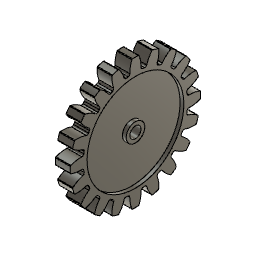
spur gear v1 (Autodesk Fusion 360 design; units mm, degrees)
Autodesk Fusion 360 part; units mm, degrees
sketch "Sketch1" plane through (0, 0, 0) normal (1, 0, 0) x (0, 1, 0)
  line L0 (0, 0) -> (0, 17.1609) construction
  line L1 (0, 0) -> (16.4802, 0) construction
  line L2 (0, 0) -> (1.095, 6.9138)
  arc A0 (0.7464, 7.1896) -> (0.4825, 8.6787) centre (-2.8935, 7.3125) ccw
  arc A1 (0.3944, 8.7411) -> (-0.3944, 8.7411) centre (0, 0) ccw
  arc A2 (0.6886, 7.9703) -> (8, 0) centre (0, 0) ccw
  arc A3 (1.095, 6.9138) -> (0.9619, 6.9336) centre (0, 0) ccw
  arc A4 (0.7464, 7.1896) -> (0.9619, 6.9336) centre (0.9963, 7.1812) ccw
  arc A5 (0.4825, 8.6787) -> (0.3944, 8.7411) centre (0.3898, 8.6412) ccw
  arc A6 (-0.3944, 8.7411) -> (-0.4825, 8.6787) centre (-0.3898, 8.6412) ccw
  arc A7 (-0.4825, 8.6787) -> (-0.7464, 7.1896) centre (2.8935, 7.3125) ccw
  arc A8 (-0.9619, 6.9336) -> (-0.7464, 7.1896) centre (-0.9963, 7.1812) ccw
  line L3 (0, 0) -> (-1.095, 6.9138)
  arc A9 (-0.9619, 6.9336) -> (-1.095, 6.9138) centre (0, 0) ccw
  dimension "d1" = 14
  dimension "d2" = 16
  dimension "d3" = 17.5
  dimension "d6" = 9
  dimension "d7" = 0.25
  dimension "d8" = 0.1
  constraint coincident L0.start L1.start
  constraint concentric A1 A3
  constraint vertical L0
  constraint perpendicular L0 L1
  constraint coincident L1 A2.end
  constraint coincident A0 A2.start
  constraint tangent A0 A4
  constraint tangent A3 A4
  constraint tangent A1 A5
  constraint tangent A0 A5
  constraint symmetric L0 L1.start L2.start
  constraint symmetric L0 A0 A7
  constraint symmetric L0 L2.end L3.end
  constraint symmetric L0 A3 A9
  constraint symmetric L0 A0.start A7.end
  constraint symmetric L0 A3.end A8.start
  constraint symmetric L0 A4 A8
  constraint symmetric L0 A1.start A1.end
  constraint symmetric L0 A0.end A6.end
  constraint symmetric L0 A5 A6
  measures "d1" diameter of A3
  measures "d2" diameter of A2
  measures "d3" diameter of A1
  measures "d6" angle of L0 L2
  measures "d7" radius of A4
  measures "d8" radius of A5
extrude "Extrude1" add sketch "Sketch1" along normal blind 2 makes body 1
pattern_circular "C-Pattern1" count 20 over 360 about axis through (1.75, 0, 0) along (1, 0, 0) of bodies 1 makes body 2 at (0.6667, -0.365, 2.3046) makes body 3 at (0, -2.72, 3.7437) makes body 4 at (0, -3.7437, 2.72) makes body 5 at (0, -4.401, 1.43) makes body 6 at (0, -4.6275, 0) makes body 7 at (0, -4.401, -1.43) makes body 8 at (0, -3.7437, -2.72) makes body 9 at (0, -2.72, -3.7437) makes body 10 at (0, -1.43, -4.401) makes body 11 at (0, 0, -4.6275) makes body 12 at (0, 1.43, -4.401) makes body 13 at (0, 2.72, -3.7437) makes body 14 at (0, 3.7437, -2.72) makes body 15 at (0, 4.401, -1.43) makes body 16 at (0, 4.6275, 0) makes body 17 at (0, 4.401, 1.43) makes body 18 at (0, 3.7437, 2.72) makes body 19 at (0, 2.72, 3.7437) makes body 20 at (0.6667, 0.365, 2.3046)
combine "Combine1" operation add target body 19 tool bodies 18 17 16 14 15 13 12 11 10 9 8 7 6 5 4 3 2 1 20
sketch "Sketch2" plane through (2, 0, 0) normal (1, 0, 0) x (0, 1, 0)
  arc A0 (5.3778, -4.8299) -> (6.7376, -5.4916) centre (7.6167, -1.9573) ccw
  arc A1 (6.7376, -5.4916) -> (6.8399, -5.4569) centre (6.7617, -5.3946) ccw
  arc A2 (6.8399, -5.4569) -> (7.3035, -4.8189) centre (0, 0) ccw
  arc A3 (7.3035, -4.8189) -> (7.3049, -4.7108) centre (7.22, -4.7638) ccw
  arc A4 (7.3049, -4.7108) -> (6.2553, -3.6221) centre (4.2152, -6.6391) ccw
  arc A5 (6.1748, -3.2972) -> (6.2553, -3.6221) centre (6.3953, -3.415) ccw
  arc A6 (6.1748, -3.2972) -> (6.297, -3.0575) centre (0, 0) ccw
  arc A7 (6.6071, -2.9316) -> (6.297, -3.0575) centre (6.5219, -3.1667) ccw
  arc A8 (6.6071, -2.9316) -> (8.1048, -3.1408) centre (7.8487, 0.4922) ccw
  arc A9 (8.1048, -3.1408) -> (8.1914, -3.0762) centre (8.0978, -3.041) ccw
  arc A10 (8.1914, -3.0762) -> (8.4351, -2.3261) centre (0, 0) ccw
  arc A11 (8.4351, -2.3261) -> (8.4031, -2.2229) centre (8.3387, -2.2995) ccw
  arc A12 (8.4031, -2.2229) -> (7.0684, -1.5118) centre (6.0604, -5.0116) ccw
  arc A13 (6.8915, -1.2277) -> (7.0684, -1.5118) centre (7.1376, -1.2716) ccw
  arc A14 (6.8915, -1.2277) -> (6.9336, -0.9619) centre (0, 0) ccw
  arc A15 (7.1896, -0.7464) -> (6.9336, -0.9619) centre (7.1812, -0.9963) ccw
  arc A16 (7.1896, -0.7464) -> (8.6787, -0.4825) centre (7.3125, 2.8935) ccw
  arc A17 (8.6787, -0.4825) -> (8.7411, -0.3944) centre (8.6412, -0.3898) ccw
  arc A18 (8.7411, -0.3944) -> (8.7411, 0.3944) centre (0, 0) ccw
  arc A19 (8.7411, 0.3944) -> (8.6787, 0.4825) centre (8.6412, 0.3898) ccw
  arc A20 (8.6787, 0.4825) -> (7.1896, 0.7464) centre (7.3125, -2.8935) ccw
  arc A21 (6.9336, 0.9619) -> (7.1896, 0.7464) centre (7.1812, 0.9963) ccw
  arc A22 (6.9336, 0.9619) -> (6.8915, 1.2277) centre (0, 0) ccw
  arc A23 (7.0684, 1.5118) -> (6.8915, 1.2277) centre (7.1376, 1.2716) ccw
  arc A24 (7.0684, 1.5118) -> (8.4031, 2.2229) centre (6.0604, 5.0116) ccw
  arc A25 (8.4031, 2.2229) -> (8.4351, 2.3261) centre (8.3387, 2.2995) ccw
  arc A26 (8.4351, 2.3261) -> (8.1914, 3.0762) centre (0, 0) ccw
  arc A27 (8.1914, 3.0762) -> (8.1048, 3.1408) centre (8.0978, 3.041) ccw
  arc A28 (8.1048, 3.1408) -> (6.6071, 2.9316) centre (7.8487, -0.4922) ccw
  arc A29 (6.297, 3.0575) -> (6.6071, 2.9316) centre (6.5219, 3.1667) ccw
  arc A30 (6.297, 3.0575) -> (6.1748, 3.2972) centre (0, 0) ccw
  arc A31 (6.2553, 3.6221) -> (6.1748, 3.2972) centre (6.3953, 3.415) ccw
  arc A32 (6.2553, 3.6221) -> (7.3049, 4.7108) centre (4.2152, 6.6391) ccw
  arc A33 (7.3049, 4.7108) -> (7.3035, 4.8189) centre (7.22, 4.7638) ccw
  arc A34 (7.3035, 4.8189) -> (6.8399, 5.4569) centre (0, 0) ccw
  arc A35 (6.8399, 5.4569) -> (6.7376, 5.4916) centre (6.7617, 5.3946) ccw
  arc A36 (6.7376, 5.4916) -> (5.3778, 4.8299) centre (7.6167, 1.9573) ccw
  arc A37 (5.044, 4.8537) -> (5.3778, 4.8299) centre (5.2241, 5.027) ccw
  arc A38 (5.044, 4.8537) -> (4.8537, 5.044) centre (0, 0) ccw
  arc A39 (4.8299, 5.3778) -> (4.8537, 5.044) centre (5.027, 5.2241) ccw
  arc A40 (4.8299, 5.3778) -> (5.4916, 6.7376) centre (1.9573, 7.6167) ccw
  arc A41 (5.4916, 6.7376) -> (5.4569, 6.8399) centre (5.3946, 6.7617) ccw
  arc A42 (5.4569, 6.8399) -> (4.8189, 7.3035) centre (0, 0) ccw
  arc A43 (4.8189, 7.3035) -> (4.7108, 7.3049) centre (4.7638, 7.22) ccw
  arc A44 (4.7108, 7.3049) -> (3.6221, 6.2553) centre (6.6391, 4.2152) ccw
  arc A45 (3.2972, 6.1748) -> (3.6221, 6.2553) centre (3.415, 6.3953) ccw
  arc A46 (3.2972, 6.1748) -> (3.0575, 6.297) centre (0, 0) ccw
  arc A47 (2.9316, 6.6071) -> (3.0575, 6.297) centre (3.1667, 6.5219) ccw
  arc A48 (2.9316, 6.6071) -> (3.1408, 8.1048) centre (-0.4922, 7.8487) ccw
  arc A49 (3.1408, 8.1048) -> (3.0762, 8.1914) centre (3.041, 8.0978) ccw
  arc A50 (3.0762, 8.1914) -> (2.3261, 8.4351) centre (0, 0) ccw
  arc A51 (2.3261, 8.4351) -> (2.2229, 8.4031) centre (2.2995, 8.3387) ccw
  arc A52 (2.2229, 8.4031) -> (1.5118, 7.0684) centre (5.0116, 6.0604) ccw
  arc A53 (1.2277, 6.8915) -> (1.5118, 7.0684) centre (1.2716, 7.1376) ccw
  arc A54 (1.2277, 6.8915) -> (0.9619, 6.9336) centre (0, 0) ccw
  arc A55 (0.7464, 7.1896) -> (0.9619, 6.9336) centre (0.9963, 7.1812) ccw
  arc A56 (0.7464, 7.1896) -> (0.4825, 8.6787) centre (-2.8935, 7.3125) ccw
  arc A57 (0.4825, 8.6787) -> (0.3944, 8.7411) centre (0.3898, 8.6412) ccw
  arc A58 (0.3944, 8.7411) -> (-0.3944, 8.7411) centre (0, 0) ccw
  arc A59 (-0.3944, 8.7411) -> (-0.4825, 8.6787) centre (-0.3898, 8.6412) ccw
  arc A60 (-0.4825, 8.6787) -> (-0.7464, 7.1896) centre (2.8935, 7.3125) ccw
  arc A61 (-0.9619, 6.9336) -> (-0.7464, 7.1896) centre (-0.9963, 7.1812) ccw
  arc A62 (-0.9619, 6.9336) -> (-1.2277, 6.8915) centre (0, 0) ccw
  arc A63 (-1.5118, 7.0684) -> (-1.2277, 6.8915) centre (-1.2716, 7.1376) ccw
  arc A64 (-1.5118, 7.0684) -> (-2.2229, 8.4031) centre (-5.0116, 6.0604) ccw
  arc A65 (-2.2229, 8.4031) -> (-2.3261, 8.4351) centre (-2.2995, 8.3387) ccw
  arc A66 (-2.3261, 8.4351) -> (-3.0762, 8.1914) centre (0, 0) ccw
  arc A67 (-3.0762, 8.1914) -> (-3.1408, 8.1048) centre (-3.041, 8.0978) ccw
  arc A68 (-3.1408, 8.1048) -> (-2.9316, 6.6071) centre (0.4922, 7.8487) ccw
  arc A69 (-3.0575, 6.297) -> (-2.9316, 6.6071) centre (-3.1667, 6.5219) ccw
  arc A70 (-3.0575, 6.297) -> (-3.2972, 6.1748) centre (0, 0) ccw
  arc A71 (-3.6221, 6.2553) -> (-3.2972, 6.1748) centre (-3.415, 6.3953) ccw
  arc A72 (-3.6221, 6.2553) -> (-4.7108, 7.3049) centre (-6.6391, 4.2152) ccw
  arc A73 (-4.7108, 7.3049) -> (-4.8189, 7.3035) centre (-4.7638, 7.22) ccw
  arc A74 (-4.8189, 7.3035) -> (-5.4569, 6.8399) centre (0, 0) ccw
  arc A75 (-5.4569, 6.8399) -> (-5.4916, 6.7376) centre (-5.3946, 6.7617) ccw
  arc A76 (-5.4916, 6.7376) -> (-4.8299, 5.3778) centre (-1.9573, 7.6167) ccw
  arc A77 (-4.8537, 5.044) -> (-4.8299, 5.3778) centre (-5.027, 5.2241) ccw
  arc A78 (-4.8537, 5.044) -> (-5.044, 4.8537) centre (0, 0) ccw
  arc A79 (-5.3778, 4.8299) -> (-5.044, 4.8537) centre (-5.2241, 5.027) ccw
  arc A80 (-5.3778, 4.8299) -> (-6.7376, 5.4916) centre (-7.6167, 1.9573) ccw
  arc A81 (-6.7376, 5.4916) -> (-6.8399, 5.4569) centre (-6.7617, 5.3946) ccw
  arc A82 (-6.8399, 5.4569) -> (-7.3035, 4.8189) centre (0, 0) ccw
  arc A83 (-7.3035, 4.8189) -> (-7.3049, 4.7108) centre (-7.22, 4.7638) ccw
  arc A84 (-7.3049, 4.7108) -> (-6.2553, 3.6221) centre (-4.2152, 6.6391) ccw
  arc A85 (-6.1748, 3.2972) -> (-6.2553, 3.6221) centre (-6.3953, 3.415) ccw
  arc A86 (-6.1748, 3.2972) -> (-6.297, 3.0575) centre (0, 0) ccw
  arc A87 (-6.6071, 2.9316) -> (-6.297, 3.0575) centre (-6.5219, 3.1667) ccw
  arc A88 (-6.6071, 2.9316) -> (-8.1048, 3.1408) centre (-7.8487, -0.4922) ccw
  arc A89 (-8.1048, 3.1408) -> (-8.1914, 3.0762) centre (-8.0978, 3.041) ccw
  arc A90 (-8.1914, 3.0762) -> (-8.4351, 2.3261) centre (0, 0) ccw
  arc A91 (-8.4351, 2.3261) -> (-8.4031, 2.2229) centre (-8.3387, 2.2995) ccw
  arc A92 (-8.4031, 2.2229) -> (-7.0684, 1.5118) centre (-6.0604, 5.0116) ccw
  arc A93 (-6.8915, 1.2277) -> (-7.0684, 1.5118) centre (-7.1376, 1.2716) ccw
  arc A94 (-6.8915, 1.2277) -> (-6.9336, 0.9619) centre (0, 0) ccw
  arc A95 (-7.1896, 0.7464) -> (-6.9336, 0.9619) centre (-7.1812, 0.9963) ccw
  arc A96 (-7.1896, 0.7464) -> (-8.6787, 0.4825) centre (-7.3125, -2.8935) ccw
  arc A97 (-8.6787, 0.4825) -> (-8.7411, 0.3944) centre (-8.6412, 0.3898) ccw
  arc A98 (-8.7411, 0.3944) -> (-8.7411, -0.3944) centre (0, 0) ccw
  arc A99 (-8.7411, -0.3944) -> (-8.6787, -0.4825) centre (-8.6412, -0.3898) ccw
  arc A100 (-8.6787, -0.4825) -> (-7.1896, -0.7464) centre (-7.3125, 2.8935) ccw
  arc A101 (-6.9336, -0.9619) -> (-7.1896, -0.7464) centre (-7.1812, -0.9963) ccw
  arc A102 (-6.9336, -0.9619) -> (-6.8915, -1.2277) centre (0, 0) ccw
  arc A103 (-7.0684, -1.5118) -> (-6.8915, -1.2277) centre (-7.1376, -1.2716) ccw
  arc A104 (-7.0684, -1.5118) -> (-8.4031, -2.2229) centre (-6.0604, -5.0116) ccw
  arc A105 (-8.4031, -2.2229) -> (-8.4351, -2.3261) centre (-8.3387, -2.2995) ccw
  arc A106 (-8.4351, -2.3261) -> (-8.1914, -3.0762) centre (0, 0) ccw
  arc A107 (-8.1914, -3.0762) -> (-8.1048, -3.1408) centre (-8.0978, -3.041) ccw
  arc A108 (-8.1048, -3.1408) -> (-6.6071, -2.9316) centre (-7.8487, 0.4922) ccw
  arc A109 (-6.297, -3.0575) -> (-6.6071, -2.9316) centre (-6.5219, -3.1667) ccw
  arc A110 (-6.297, -3.0575) -> (-6.1748, -3.2972) centre (0, 0) ccw
  arc A111 (-6.2553, -3.6221) -> (-6.1748, -3.2972) centre (-6.3953, -3.415) ccw
  arc A112 (-6.2553, -3.6221) -> (-7.3049, -4.7108) centre (-4.2152, -6.6391) ccw
  arc A113 (-7.3049, -4.7108) -> (-7.3035, -4.8189) centre (-7.22, -4.7638) ccw
  arc A114 (-7.3035, -4.8189) -> (-6.8399, -5.4569) centre (0, 0) ccw
  arc A115 (-6.8399, -5.4569) -> (-6.7376, -5.4916) centre (-6.7617, -5.3946) ccw
  arc A116 (-6.7376, -5.4916) -> (-5.3778, -4.8299) centre (-7.6167, -1.9573) ccw
  arc A117 (-5.044, -4.8537) -> (-5.3778, -4.8299) centre (-5.2241, -5.027) ccw
  arc A118 (-5.044, -4.8537) -> (-4.8537, -5.044) centre (0, 0) ccw
  arc A119 (-4.8299, -5.3778) -> (-4.8537, -5.044) centre (-5.027, -5.2241) ccw
  arc A120 (-4.8299, -5.3778) -> (-5.4916, -6.7376) centre (-1.9573, -7.6167) ccw
  arc A121 (-5.4916, -6.7376) -> (-5.4569, -6.8399) centre (-5.3946, -6.7617) ccw
  arc A122 (-5.4569, -6.8399) -> (-4.8189, -7.3035) centre (0, 0) ccw
  arc A123 (-4.8189, -7.3035) -> (-4.7108, -7.3049) centre (-4.7638, -7.22) ccw
  arc A124 (-4.7108, -7.3049) -> (-3.6221, -6.2553) centre (-6.6391, -4.2152) ccw
  arc A125 (-3.2972, -6.1748) -> (-3.6221, -6.2553) centre (-3.415, -6.3953) ccw
  arc A126 (-3.2972, -6.1748) -> (-3.0575, -6.297) centre (0, 0) ccw
  arc A127 (-2.9316, -6.6071) -> (-3.0575, -6.297) centre (-3.1667, -6.5219) ccw
  arc A128 (-2.9316, -6.6071) -> (-3.1408, -8.1048) centre (0.4922, -7.8487) ccw
  arc A129 (-3.1408, -8.1048) -> (-3.0762, -8.1914) centre (-3.041, -8.0978) ccw
  arc A130 (-3.0762, -8.1914) -> (-2.3261, -8.4351) centre (0, 0) ccw
  arc A131 (-2.3261, -8.4351) -> (-2.2229, -8.4031) centre (-2.2995, -8.3387) ccw
  arc A132 (-2.2229, -8.4031) -> (-1.5118, -7.0684) centre (-5.0116, -6.0604) ccw
  arc A133 (-1.2277, -6.8915) -> (-1.5118, -7.0684) centre (-1.2716, -7.1376) ccw
  arc A134 (-1.2277, -6.8915) -> (-0.9619, -6.9336) centre (0, 0) ccw
  arc A135 (-0.7464, -7.1896) -> (-0.9619, -6.9336) centre (-0.9963, -7.1812) ccw
  arc A136 (-0.7464, -7.1896) -> (-0.4825, -8.6787) centre (2.8935, -7.3125) ccw
  arc A137 (-0.4825, -8.6787) -> (-0.3944, -8.7411) centre (-0.3898, -8.6412) ccw
  arc A138 (-0.3944, -8.7411) -> (0.3944, -8.7411) centre (0, 0) ccw
  arc A139 (0.3944, -8.7411) -> (0.4825, -8.6787) centre (0.3898, -8.6412) ccw
  arc A140 (0.4825, -8.6787) -> (0.7464, -7.1896) centre (-2.8935, -7.3125) ccw
  arc A141 (0.9619, -6.9336) -> (0.7464, -7.1896) centre (0.9963, -7.1812) ccw
  arc A142 (0.9619, -6.9336) -> (1.2277, -6.8915) centre (0, 0) ccw
  arc A143 (1.5118, -7.0684) -> (1.2277, -6.8915) centre (1.2716, -7.1376) ccw
  arc A144 (1.5118, -7.0684) -> (2.2229, -8.4031) centre (5.0116, -6.0604) ccw
  arc A145 (2.2229, -8.4031) -> (2.3261, -8.4351) centre (2.2995, -8.3387) ccw
  arc A146 (2.3261, -8.4351) -> (3.0762, -8.1914) centre (0, 0) ccw
  arc A147 (3.0762, -8.1914) -> (3.1408, -8.1048) centre (3.041, -8.0978) ccw
  arc A148 (3.1408, -8.1048) -> (2.9316, -6.6071) centre (-0.4922, -7.8487) ccw
  arc A149 (3.0575, -6.297) -> (2.9316, -6.6071) centre (3.1667, -6.5219) ccw
  arc A150 (3.0575, -6.297) -> (3.2972, -6.1748) centre (0, 0) ccw
  arc A151 (3.6221, -6.2553) -> (3.2972, -6.1748) centre (3.415, -6.3953) ccw
  arc A152 (3.6221, -6.2553) -> (4.7108, -7.3049) centre (6.6391, -4.2152) ccw
  arc A153 (4.7108, -7.3049) -> (4.8189, -7.3035) centre (4.7638, -7.22) ccw
  arc A154 (4.8189, -7.3035) -> (5.4569, -6.8399) centre (0, 0) ccw
  arc A155 (5.4569, -6.8399) -> (5.4916, -6.7376) centre (5.3946, -6.7617) ccw
  arc A156 (5.4916, -6.7376) -> (4.8299, -5.3778) centre (1.9573, -7.6167) ccw
  arc A157 (4.8537, -5.044) -> (4.8299, -5.3778) centre (5.027, -5.2241) ccw
  arc A158 (4.8537, -5.044) -> (5.044, -4.8537) centre (0, 0) ccw
  arc A159 (5.3778, -4.8299) -> (5.044, -4.8537) centre (5.2241, -5.027) ccw
  circle A160 centre (0, 0) radius 6.5
  circle A161 centre (0, 0) radius 0.75
  circle A162 centre (0, 0) radius 1.25
  dimension "d13" = 13
  dimension "d14" = 1.5
  dimension "d15" = 2.5
  constraint coincident A2.centre A6.centre
  constraint concentric A160 A161
  constraint concentric A160 A162
  measures "d13" diameter of A160
  measures "d14" diameter of A161
  measures "d15" diameter of A162
extrude "Extrude2" cut sketch "Sketch2" against normal blind 0.5 contours A160 bodies 19
extrude "Extrude3" cut sketch "Sketch2" against normal blind 7.916 contours A161 bodies 19
